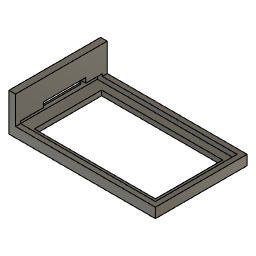
sdr3 (Autodesk Fusion 360 design; units mm, degrees)
Autodesk Fusion 360 part; units mm, degrees
sketch "Sketch1" plane through (0, 0, 0) normal (0, 0, 1) x (1, 0, 0)
  line L0 (0, 0) -> (42, 0)
  line L1 (42, 0) -> (42, 24.4)
  line L2 (42, 24.4) -> (0, 24.4)
  line L3 (0, 24.4) -> (0, 0)
  line L4 (-0.2, 24.6) -> (42.2, 24.6)
  line L5 (42.2, 24.6) -> (42.2, -0.2)
  line L6 (42.2, -0.2) -> (-0.2, -0.2)
  line L7 (-0.2, -0.2) -> (-0.2, 24.6)
  line L8 (-0.7, 26.1) -> (43.7, 26.1)
  line L9 (43.7, 26.1) -> (43.7, -1.7)
  line L10 (43.7, -1.7) -> (-0.7, -1.7)
  line L11 (-0.7, -1.7) -> (-0.7, 26.1)
  line L12 (-0.7, 26.1) -> (1.3, 26.1)
  line L13 (1.3, 26.1) -> (1.3, -1.7)
  line L14 (1.3, -1.7) -> (-0.7, -1.7)
  line L15 (-0.7, -1.7) -> (-0.7, 26.1)
  line L16 (3.3, 22.4) -> (40, 22.4)
  line L17 (40, 22.4) -> (40, 2)
  line L18 (40, 2) -> (3.3, 2)
  line L19 (3.3, 2) -> (3.3, 22.4)
  dimension "d1" = 42
  dimension "d2" = 24.4
  dimension "d3" = 0.2
  dimension "d4" = 0.2
  dimension "d5" = 0.2
  dimension "d6" = 0.2
  dimension "d7" = 0.5
  dimension "d8" = 1.5
  dimension "d9" = 1.5
  dimension "d10" = 1.5
  dimension "d11" = 2
  dimension "d12" = 27.8
  dimension "d13" = 2
  dimension "d14" = 2
  dimension "d15" = 2
  dimension "d16" = 2
  constraint horizontal L0
  constraint vertical L1
  constraint horizontal L2
  constraint vertical L3
  constraint coincident L0.start L3.end
  constraint horizontal L4
  constraint vertical L5
  constraint horizontal L6
  constraint vertical L7
  constraint horizontal L8
  constraint vertical L9
  constraint horizontal L10
  constraint vertical L11
  constraint horizontal L12
  constraint vertical L13
  constraint horizontal L14
  constraint vertical L15
  constraint horizontal L16
  constraint vertical L17
  constraint horizontal L18
  constraint vertical L19
  measures "d1" distance of L0.start L0.end
  measures "d2" distance of L0.start L2.end
  measures "d3" distance of L3 L7
  measures "d4" distance of L2 L4
  measures "d5" distance of L0 L6
  measures "d6" distance of L1 L5
  measures "d7" distance of L7 L11
  measures "d8" distance of L4 L8
  measures "d9" distance of L6 L10
  measures "d10" distance of L5 L9
  measures "d11" distance of L8.start L12.end
  measures "d12" distance of L8.start L10.end
  measures "d13" distance of L13 L19
  measures "d14" distance of L2 L16
  measures "d15" distance of L0 L18
  measures "d16" distance of L1 L17
extrude "Extrude1" add sketch "Sketch1" against normal blind 1.5
extrude "Extrude2" add sketch "Sketch1" along normal blind 1.5 contours L4 L5 L6 L8 L9 L10 L13
extrude "Extrude3" add sketch "Sketch1" along normal blind 10 contours L4 L6 L7 L8 L10 L11 L12 L13 L14 L15
sketch "Sketch2" plane through (-0.7, 0, 0) normal (-1, 0, 0) x (0, -1, 0)
  line L0 (-26.1, 10) -> (-26.1, -1.5)
  line L1 (-26.1, -1.5) -> (1.7, -1.5)
  line L2 (1.7, -1.5) -> (1.7, 10)
  line L3 (1.7, 10) -> (-26.1, 10)
  line L4 (-24.4, 0) -> (0, 0)
  line L5 (0, 0) -> (0, 1.2)
  line L6 (0, 1.2) -> (-24.4, 1.2)
  line L7 (-24.4, 1.2) -> (-24.4, 0)
  line L8 (-19.6, 1.2) -> (-4.8, 1.2)
  line L9 (-4.8, 1.2) -> (-4.8, 3.2)
  line L10 (-4.8, 3.2) -> (-19.6, 3.2)
  line L11 (-19.6, 3.2) -> (-19.6, 1.2)
  line L12 (-4.8, 3.2) -> (-6.8, 3.2)
  line L13 (-6.8, 3.2) -> (-6.8, 1.2)
  line L14 (-6.8, 1.2) -> (-4.8, 1.2)
  line L15 (-4.8, 1.2) -> (-4.8, 3.2)
  circle A0 centre (-13.2, 3.2) radius 6.4
  dimension "d23" = 24.4
  dimension "d24" = 1.2
  dimension "d25" = 1.7
  dimension "d26" = 14.8
  dimension "d27" = 2
  dimension "d28" = 4.8
  dimension "d29" = 2
  dimension "d30" = 2
  dimension "d31" = 12.8
  dimension "d32" = 6.4
  constraint horizontal L4
  constraint vertical L5
  constraint horizontal L6
  constraint vertical L7
  constraint horizontal L8
  constraint vertical L9
  constraint horizontal L10
  constraint vertical L11
  constraint coincident L6 L8.start
  constraint horizontal L12
  constraint vertical L13
  constraint horizontal L14
  constraint vertical L15
  constraint coincident L10 A0.centre
  measures "d23" distance of L4.start L4.end
  measures "d24" distance of L4.start L6.end
  measures "d25" distance of L0 L7
  measures "d26" distance of L8.start L8.end
  measures "d27" distance of L8.start L10.end
  measures "d28" distance of L7 L11
  measures "d29" distance of L9.end L12.end
  measures "d30" distance of L9.end L8.end
  measures "d31" diameter of A0
  measures "d32" distance of L11 A0.centre
extrude "Extrude4" add sketch "Sketch2" against normal blind 2 contours L0 L1 L2 L3 L4 L5 L6 L7 L9 L10 L11 L12 L15 A0 | L1 L4 A0 | L10 A0 | L6 L8 L9 L10 L12 L13 L14 L15
extrude "Extrude5" cut sketch "Sketch2" against normal blind 1 contours L6 L8 L10 A0 | L6 L8 L11 A0 | L6 L8 L13 A0 | L10 A0
extrude "Extrude6" cut 1 faces at (0.3, 24.4, 0.8) along direction (0, 1, 0) blind 0.2
extrude "Extrude7" cut 1 faces at (0.3, 0, 0.4) along direction (0, -1, 0) blind 0.2
extrude "Extrude8" cut 2 faces at (0.8, 4.4667, 1.2) (0.8, 22.9333, 1.2) along direction (0, 0, 1) blind 0.5
extrude "Extrude9" cut 1 faces at (0.9667, 11.0667, 3.2) along direction (0, 0, 1) blind 0.5
extrude "Extrude10" cut 2 faces at (0.8, 4.4667, 1.7) (0.8, 22.9333, 1.7) along direction (0, 0, 1) blind 0.5
equation "d25 = ( 3.4 / 2 ) * 1 mm"
equation "d28 = ( 9.6 / 2 ) * 1 mm"
